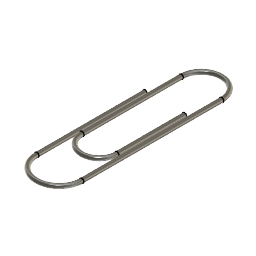
Paperclip (Autodesk Fusion 360 design; units mm, degrees)
part number: 2026-08-05-22-10-43-632
Autodesk Fusion 360 part; units mm, degrees
sketch "Sketch3" plane through (0, 0, 0) normal (0, 0, 1) x (1, 0, 0)
  line L0 (-2.5, 0) -> (-2.5, -24)
  arc A0 (-2.5, -24) -> (7.5, -24) centre (2.5, -24) ccw
  line L1 (7.5, -24) -> (7.5, 7)
  arc A1 (7.5, 7) -> (-1.5, 7) centre (3, 7) ccw
  line L2 (-1.5, 7) -> (-1.5, -15)
  arc A2 (-1.5, -15) -> (6.3, -15) centre (2.4, -15) ccw
  line L3 (6.3, -15) -> (6.3, 0)
  dimension "d21" = 24
  dimension "d22" = 5
  dimension "d23" = 31
  dimension "d24" = 4.5
  dimension "d25" = 22
  dimension "d26" = 3.9
  dimension "d27" = 15
  constraint vertical L0
  constraint tangent L0 A0
  constraint vertical L1
  constraint tangent L1 A1
  constraint vertical L2
  constraint tangent L2 A2
  constraint vertical L3
  measures "d21" distance of L0.start L0.end
  measures "d22" radius of A0
  measures "d23" distance of A0.end L1.end
  measures "d24" radius of A1
  measures "d25" distance of A1.end L2.end
  measures "d26" radius of A2
  measures "d27" distance of A2.end L3.end
sketch "Sketch4" plane through (0, 0, 0) normal (0, 1, 0) x (1, 0, 0)
  circle A0 centre (-2.4732, 0.0221) radius 0.5
  dimension "d28" = 1
  measures "d28" diameter of A0
sweep "Sweep1" add profiles "Sketch4" path "Sketch3" along L0 A0 L1 A1 L2 A2 L3 section 1
